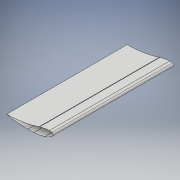
# Autodesk Inventor part: GFRP_main
Saved by Autodesk Inventor 2018.2 (Build 222227000, 227)
## iProperties
Created: 2018-04-22
Part Number: GFRP_main
Material: 一般
Document SubType Name: Modeling
Designer: ku_sk
Density: 1 g/cm^3
Appearance: 既定
Author: ku_sk
Autodesk Inventor part; units mm, degrees
ref_plane "YZ Plane" through (0, 0, 0) normal (1, 0, 0) x (0, 1, 0)
ref_plane "XZ Plane" through (0, 0, 0) normal (0, 1, 0) x (-1, 0, 0)
ref_plane "XY Plane" through (0, 0, 0) normal (0, 0, 1) x (1, 0, 0)
sketch "スケッチ1" plane through (0, 0, 0) normal (0, 1, 0) x (-1, 0, 0)
  arc A0 (182.3045, -62.8657) -> (348.4892, -47.2216) centre (162.2533, 1040.6287) ccw projected
  arc A1 (135.2834, -62.3282) -> (182.3045, -62.8657) centre (167.871, 731.467) ccw projected
  arc A2 (49.3906, -47.0603) -> (135.2834, -62.3282) centre (148.588, 261.756) ccw projected
  arc A3 (0.1309, -22.8654) -> (49.3906, -47.0603) centre (107.173, 132.825) ccw projected
  arc A4 (-13.3538, -9.7713) -> (0.1309, -22.8654) centre (31.9, 23.342) ccw projected
  arc A5 (-7.3318, 8.7424) -> (-13.3538, -9.7713) centre (-3.6695, -2.6851) ccw projected
  arc A6 (12.9042, 11.391) -> (-7.3318, 8.7424) centre (10.0641, -45.5382) ccw projected
  arc A7 (90.1175, -2.8524) -> (12.9042, 11.391) centre (-1.8944, -285.2401) ccw projected
  arc A8 (90.1175, -2.8524) -> (94.8834, -4.3943) centre (462.8125, 1140.9603) ccw projected
  arc A9 (94.8834, -4.3943) -> (348.3291, -45.236) centre (355.7675, 807.7316) ccw projected
  arc A10 (348.4892, -47.2216) -> (348.3291, -45.236) centre (348.3204, -46.2359) ccw projected
  circle A11 centre (29.3651, -6.1392) radius 6 projected
  circle A12 centre (239.8151, -50.1371) radius 6 projected
  point P0 (0, 0)
extrude "押し出し1" add sketch "スケッチ1" along normal mid plane 946 contours A1 A2 A3 A4 A5 A6 A7 A8 A9 A10 A0 | A11 | A12
shell "シェル1" thickness 1 outward yes removed faces 2 at (-105.6232, -473, -25.6277) at (-105.6232, 473, -25.6277)
